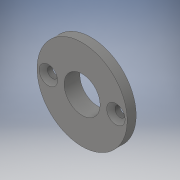
# Autodesk Inventor part: Крышка
Saved by Autodesk Inventor 2019.3 (Build 233278000, 278)
## iProperties
Created: 2020-04-02
Part Number: Крышка
Material: Типовые
Document SubType Name: Modeling
Designer: Admin
Density: 1 g/cm^3
Appearance: По умолчанию
Mass: 60.8674 g
Surface Area: 150.863 cm^2
Volume: 60.8674 cm^3
Author: Admin
Autodesk Inventor part; units mm, degrees
ref_plane "YZ Plane" through (0, 0, 0) normal (1, 0, 0) x (0, 1, 0)
ref_plane "XZ Plane" through (0, 0, 0) normal (0, 1, 0) x (-1, 0, 0)
ref_plane "XY Plane" through (0, 0, 0) normal (0, 0, 1) x (1, 0, 0)
sketch "Эскиз1" plane through (0, 0, 0) normal (0, 0, 1) x (1, 0, 0)
  circle A0 centre (0, 0) radius 40
  dimension "d0" = 80
  constraints: 1 centre point, 1 coincident
  measures "d0" diameter of A0
extrude "Выдавливание1" add sketch "Эскиз1" along normal blind 8
sketch "Эскиз2" plane through (0, 0, 0) normal (0, 0, -1) x (-1, 0, 0)
  circle A0 centre (0, 0) radius 22
  dimension "d3" = 44
  constraints: 1 centre point, 1 coincident
  measures "d3" diameter of A0
extrude "Выдавливание2" add sketch "Эскиз2" along normal blind 6
sketch "Эскиз3" plane through (0, 0, -6) normal (0, 0, -1) x (-1, 0, 0)
  circle A0 centre (0, 0) radius 16
  dimension "d6" = 32
  constraints: 1 centre point, 1 coincident
  measures "d6" diameter of A0
extrude "Выдавливание3" cut sketch "Эскиз3" against normal through all
chamfer "Фаска1" distance 2 angle 45 1 edges at (22, 0, -6)
sketch "Эскиз4" plane through (0, 0, 8) normal (0, 0, 1) x (1, 0, 0)
  point P0 (0, 0)
  point P1 (-30, 0)
  point P2 (30, 0)
  dimension "d12" = 30
  dimension "d13" = 60
  constraints: 2 horizontal alignment
  measures "d12" distance of point (0, 0) point (-30, 0)
  measures "d13" distance of point (30, 0) point (-30, 0)
hole "Отверстие1" at (-30, 0, 8) at (30, 0, 8) direction (0, 0, -1) diameter 9 end through all countersink diameter 16.4 countersink angle 90 clearance for "Винт крепежный с плоской головкой" size "M8" standard "ANSI метрическая"
